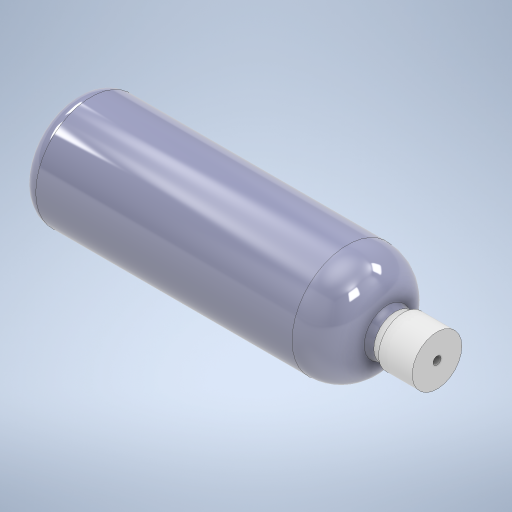
# Autodesk Inventor part: petbottle_hn
Saved by Autodesk Inventor 2024 (Build 280153000, 153)
## iProperties
Created: 2020-03-23
Part Number: petbottle_hn
Material: 一般
Document SubType Name: Modeling
Designer: Haruka
Density: 1 g/cm^3
Appearance: 既定
Author: Haruka
Autodesk Inventor part; units mm, degrees
ref_plane "YZ Plane" through (0, 0, 0) normal (1, 0, 0) x (0, 1, 0)
ref_plane "XZ Plane" through (0, 0, 0) normal (0, 1, 0) x (-1, 0, 0)
ref_plane "XY Plane" through (0, 0, 0) normal (0, 0, 1) x (1, 0, 0)
sketch "スケッチ1" plane through (0, 0, 0) normal (0, 1, 0) x (-1, 0, 0)
  line L0 (0, 0) -> (160, 0)
  line L1 (160, 0) -> (160, -34.5)
  line L2 (160, -34.5) -> (0, -34.5)
  line L3 (0, -34.5) -> (0, 0)
  line L4 (160, 0) -> (170, 0)
  line L5 (170, 0) -> (170, -24.5)
  arc A0 (160, -34.5) -> (170, -24.5) centre (160, -24.5) ccw
  line L6 (0, -34.5) -> (0, -14.5)
  line L7 (0, -14.5) -> (-25, -14.5)
  line L8 (-25, -14.5) -> (-25, 0)
  line L9 (-25, 0) -> (-30, 0)
  line L10 (-30, 0) -> (-30, -13.5)
  arc A1 (-25, -14.5) -> (-30, -13.5) centre (-29.2733, -22.8663) ccw
  arc A2 (-25, -14.5) -> (0, -34.5) centre (0, -8.875) ccw
  line L11 (-30, -13.5) -> (-35, -13.5)
  line L12 (-35, -13.5) -> (-35, 0)
  line L13 (-35, 0) -> (-30, 0)
  line L14 (-30, 0) -> (-30, -13.5)
  line L15 (-35, 0) -> (-35, -15.5)
  line L16 (-35, -15.5) -> (-56, -15.5)
  line L17 (-56, -15.5) -> (-56, 0)
  line L18 (-56, 0) -> (-35, 0)
  line L19 (-35, 0) -> (-35, -15.5)
  line L20 (0, 0) -> (-25, 0)
  point P0 (-35, 0)
  dimension "d0" = 160
  dimension "d1" = 34.5
  dimension "d2" = 10
  dimension "d3" = 24.5
  dimension "d4" = 20
  dimension "d5" = 25
  dimension "d7" = 5
  dimension "d8" = 13.5
  dimension "d9" = 9.3945
  dimension "d10" = 5
  dimension "d11" = 15.5
  dimension "d12" = 21
  constraints: 42 end point, 6 parallel, 6 point on circle, 5 horizontal, 4 perpendicular, 4 vertical, 3 centre point, 2 tangent, 1 collinear, 1 point on line
  measures "d0" distance of L1.end L2.end
  measures "d1" distance of L0.end L1.end
  measures "d2" distance of L0.end L4.end
  measures "d3" distance of L4.end L5.end
  measures "d4" distance of L2.end L6.end
  measures "d5" distance of L6.end L7.end
  measures "d7" distance of L8.end L9.end
  measures "d8" distance of L9.end L10.end
  measures "d9" radius of A1
  measures "d10" distance of L12.end L13.end
  measures "d11" distance of L12.end L15.end
  measures "d12" distance of L17.end L18.end
revolve "回転1" add sketch "スケッチ1" angle 360 about axis through (0, 0, 0) along (-1, 0, 0)
sketch "スケッチ2" plane through (56, 0, 0) normal (1, 0, 0) x (0, 0, -1)
  circle A0 centre (0, 0) radius 13.5 projected
  constraints: 1 coincident
hole "穴1" at (56, 0, 0) direction (-1, 0, 0) diameter 5 depth 5
